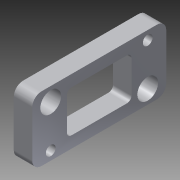
# Autodesk Inventor part: M - Carriage Plate Part 1
Saved by Autodesk Inventor 2013 (Build 170138000, 138)
## iProperties
Created: 2013-02-17
Part Number: M - Carriage Plate Part 1
Material: Aluminum 6061
Document SubType Name: Modeling
Designer: Moses
Mass: 82.7474 g
Surface Area: 116.026 cm^2
Volume: 30.5341 cm^3
Density: 2.71 g/cm^3
Author: Moses
Autodesk Inventor part; units mm, degrees
ref_plane "YZ Plane" through (0, 0, 0) normal (1, 0, 0) x (0, 1, 0)
ref_plane "XZ Plane" through (0, 0, 0) normal (0, 1, 0) x (-1, 0, 0)
ref_plane "XY Plane" through (0, 0, 0) normal (0, 0, 1) x (1, 0, 0)
sketch "Sketch1" plane through (0, 0, 0) normal (1, 0, 0) x (0, 1, 0)
  line L0 (0, 0) -> (44.45, 0)
  line L1 (44.45, 0) -> (44.45, 92.075)
  line L2 (44.45, 92.075) -> (0, 92.075)
  line L3 (0, 92.075) -> (0, 0)
  line L4 (14.2875, 92.075) -> (14.2875, 0) construction
  line L5 (30.1625, 92.075) -> (30.1625, 0) construction
  line L6 (22.225, 92.075) -> (22.225, 0) construction
  circle A0 centre (34.925, 79.375) radius 4.7625 construction
  circle A1 centre (9.525, 12.7) radius 4.7625 construction
  circle A2 centre (34.925, 79.375) radius 7.1437
  circle A3 centre (9.525, 12.7) radius 7.1437
  line L7 (7.9375, 68.2625) -> (36.5125, 68.2625)
  line L8 (36.5125, 68.2625) -> (36.5125, 23.8125)
  line L9 (36.5125, 23.8125) -> (7.9375, 23.8125)
  line L10 (7.9375, 23.8125) -> (7.9375, 68.2625)
  line L11 (7.9375, 46.0375) -> (36.5125, 46.0375) construction
  circle A4 centre (6.0325, 79.375) radius 3.3782
  circle A5 centre (38.4175, 12.7) radius 3.3782
  point P0 (22.225, 68.2625)
  point P1 (22.225, 46.0375)
  dimension "d0" = 15.875
  dimension "d2" = 7.9375
  dimension "d3" = 44.45
  dimension "d4" = 9.525
  dimension "d5" = 9.525
  dimension "d6" = 92.075
  dimension "d7" = 12.7
  dimension "d8" = 12.7
  dimension "d11" = 14.2875
  dimension "d12" = 14.2875
  dimension "d15" = 28.575
  dimension "d16" = 44.45
  dimension "d19" = 6.7564
  dimension "d20" = 6.7564
  dimension "d21" = 8.255
  dimension "d22" = 12.7
  dimension "d23" = 8.255
  dimension "d24" = 12.7
  constraints: 24 end point, 7 midpoint, 6 centre point, 5 parallel, 5 point on line, 3 perpendicular, 2 coincident, 2 horizontal, 2 tangent
  measures "d0" distance between parallel lines of L5 L4
  measures "d2" distance between parallel lines of L5 L6
  measures "d3" distance of L1.end L2.end
  measures "d4" diameter of A0
  measures "d5" diameter of A1
  measures "d6" distance of L2.end L0.start
  measures "d7" distance from line of L2 A0.centre
  measures "d8" distance from line of L0 A1.centre
  measures "d11" diameter of A2
  measures "d12" diameter of A3
  measures "d15" distance of L7.start L7.end
  measures "d16" distance of L9.end L7.start
  measures "d19" diameter of A4
  measures "d20" diameter of A5
  measures "d21" distance from line of L4 A4.centre
  measures "d22" distance from line of L2 A4.centre
  measures "d23" distance from line of A5.centre L5
  measures "d24" distance from line of L0 A5.centre
extrude "Extrusion1" add sketch "Sketch1" along normal blind 12.7
fillet "Fillet1" radius 6.35 4 edges at (6.35, 0, 92.075) (6.35, 44.45, 92.075) (6.35, 0, 0) (6.35, 44.45, 0)
fillet "Fillet1" radius 3.175 4 edges at (6.35, 7.9375, 68.2625) (6.35, 36.5125, 68.2625) (6.35, 36.5125, 23.8125) (6.35, 7.9375, 23.8125)
equation "\"d2\" = 0.5 * d0"
equation "\"d23\" = d21"
body "Solid1"
